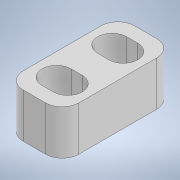
# Autodesk Inventor part: Part148
Saved by Autodesk Inventor 2021.3 (Build 253353000, 353)
## iProperties
Created: 2021-06-26
Part Number: Part148
Material: Generic
Document SubType Name: Modeling
Designer: Fabijan_Sven
Density: 1 g/cm^3
Appearance: Default
Author: Fabijan_Sven
Autodesk Inventor part; units mm, degrees
ref_plane "YZ Plane" through (0, 0, 0) normal (1, 0, 0) x (0, 1, 0)
ref_plane "XZ Plane" through (0, 0, 0) normal (0, 1, 0) x (-1, 0, 0)
ref_plane "XY Plane" through (0, 0, 0) normal (0, 0, 1) x (1, 0, 0)
sketch "Sketch1" plane through (0, 0, 0) normal (0, 1, 0) x (-1, 0, 0)
  line L0 (0, 0) -> (10, 0)
  line L1 (10, 0) -> (10, -20)
  line L2 (10, -20) -> (0, -20)
  line L3 (0, -20) -> (0, 0)
  arc A0 (5, -7.4) -> (6, -7.6) centre (6, -5) ccw
  arc A1 (5, -2.6) -> (4, -2.4) centre (4, -5) ccw
  line L4 (4, -2.4) -> (6, -2.4)
  line L5 (6, -2.4) -> (6, -3.3387)
  line L6 (6, -7.6) -> (4, -7.6)
  line L7 (4, -7.6) -> (4, -2.4)
  arc A2 (6, -3.3387) -> (5, -2.6) centre (4, -5) ccw
  line L8 (6, -3.3387) -> (6, -7.6)
  arc A3 (4, -2.4) -> (6, -3.3387) centre (4, -5) ccw
  arc A4 (6, -2.4) -> (5, -2.6) centre (6, -5) ccw
  arc A5 (6, -7.6) -> (6, -2.4) centre (6, -5) ccw
  line L9 (11.1663, -10) -> (-5.9269, -10) construction
  arc A6 (6, -12.4) -> (5, -12.6) centre (6, -15) ccw
  arc A7 (4, -17.6) -> (5, -17.4) centre (4, -15) ccw
  line L10 (4, -17.6) -> (6, -17.6)
  line L11 (6, -17.6) -> (6, -16.6613)
  line L12 (6, -12.4) -> (4, -12.4)
  line L13 (4, -12.4) -> (4, -17.6)
  arc A8 (5, -17.4) -> (6, -16.6613) centre (4, -15) ccw
  line L14 (6, -16.6613) -> (6, -12.4)
  arc A9 (6, -16.6613) -> (4, -17.6) centre (4, -15) ccw
  arc A10 (5, -17.4) -> (6, -17.6) centre (6, -15) ccw
  arc A11 (6, -17.6) -> (6, -12.4) centre (6, -15) ccw
  dimension "d0" = 20
  dimension "d1" = 10
  dimension "d2" = 5.2
  dimension "d3" = 5.2
  dimension "d4" = 5
  dimension "d5" = 5
  dimension "d6" = 4
  dimension "d7" = 4
  dimension "d8" = 10
  constraints: 30 end point, 30 point on circle, 12 centre point, 9 symmetric about line, 5 parallel, 3 horizontal, 3 perpendicular, 6 other
  measures "d0" distance of L0.end L1.end
  measures "d1" distance of L1.end L2.end
  measures "d2" diameter of A0
  measures "d3" diameter of A1
  measures "d4" distance from line of L0 A0.centre
  measures "d5" distance from line of L0 A1.centre
  measures "d6" distance from line of A0.centre L1
  measures "d7" distance from line of L3 A1.centre
  measures "d8" distance between parallel lines of L0 L9
extrude "Extrusion1" add sketch "Sketch1" along normal blind 8
fillet "Fillet1" radius 3 4 edges at (0, 4, 0) (0, 4, -20) (-10, 4, -20) (-10, 4, 0)
body "Solid1"
